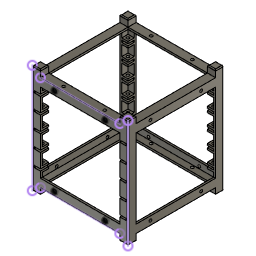
сборка кубсата (Autodesk Fusion 360 archive; units mm, degrees)
design "кубсат 3"
Autodesk Fusion 360 part; units mm, degrees
(part 1 of 2)
sketch "Sketch1" plane through (0, 0, 0) normal (0, 0, 1) x (1, 0, 0)
  line L0 (0, 0) -> (8.5, 0)
  line L1 (8.5, 0) -> (8.5, 8.5)
  line L2 (8.5, 8.5) -> (0, 8.5)
  line L3 (0, 8.5) -> (0, 0)
  line L4 (0, 100) -> (8.5, 100)
  line L5 (8.5, 100) -> (8.5, 91.5)
  line L6 (8.5, 91.5) -> (0, 91.5)
  line L7 (0, 91.5) -> (0, 100)
  line L8 (100, 100) -> (91.5, 100)
  line L9 (91.5, 100) -> (91.5, 91.5)
  line L10 (91.5, 91.5) -> (100, 91.5)
  line L11 (100, 91.5) -> (100, 100)
  line L12 (100, 0) -> (91.5, 0)
  line L13 (91.5, 0) -> (91.5, 8.5)
  line L14 (91.5, 8.5) -> (100, 8.5)
  line L15 (100, 8.5) -> (100, 0)
  dimension "d1" = 100
  dimension "d2" = 100
  dimension "d3" = 8.5
  dimension "d4" = 8.5
  dimension "d5" = 8.5
  dimension "d6" = 8.5
  dimension "d7" = 8.5
  dimension "d8" = 8.5
  dimension "d9" = 83
  dimension "d10" = 83
  dimension "d11" = 8.5
  dimension "d12" = 8.5
  constraint horizontal L0
  constraint vertical L1
  constraint horizontal L2
  constraint vertical L3
  constraint coincident L0.start L3.end
  constraint horizontal L4
  constraint vertical L5
  constraint horizontal L6
  constraint vertical L7
  constraint horizontal L8
  constraint vertical L9
  constraint horizontal L10
  constraint vertical L11
  constraint horizontal L12
  constraint vertical L13
  constraint horizontal L14
  constraint vertical L15
  measures "d1" distance of L0.start L12.start
  measures "d2" distance of L0.start L4.start
  measures "d3" distance of L0.start L0.end
  measures "d4" distance of L0.start L2.end
  measures "d5" distance of L4.start L6.end
  measures "d6" distance of L8.start L8.end
  measures "d7" distance of L12.start L12.end
  measures "d8" distance of L12.start L14.end
  measures "d9" distance of L5 L9
  measures "d10" distance of L10 L14
  measures "d11" distance of L8.start L10.end
  measures "d12" distance of L4.start L4.end
extrude "Extrude1" add sketch "Sketch1" along normal blind 113.5 makes body 1 at (0, 5.6667, 37.8333) makes body 2 at (100, 94.3333, 37.8333) makes body 3 at (2.8333, 100, 37.8333) makes body 4 at (97.1667, 0, 37.8333)
ref_plane "WorkPlane1" through (4.25, 91.5, 56.75) normal (0, -1, 0) x (1, 0, 0)
sketch "Sketch2" plane through (4.25, 91.5, 56.75) normal (0, -1, 0) x (1, 0, 0)
  line L0 (4.25, 47.75) -> (-4.25, 47.75)
  line L1 (-4.25, 47.75) -> (-4.25, 49.75)
  line L2 (-4.25, 49.75) -> (4.25, 49.75)
  line L3 (4.25, 49.75) -> (4.25, 47.75)
  line L4 (-4.25, 56.75) -> (4.25, 56.75)
  line L5 (-4.25, -56.75) -> (-4.25, 56.75)
  line L6 (-4.25, -47.75) -> (4.25, -47.75)
  line L7 (4.25, -47.75) -> (4.25, -49.75)
  line L8 (4.25, -49.75) -> (-4.25, -49.75)
  line L9 (-4.25, -49.75) -> (-4.25, -47.75)
  line L10 (4.25, -56.75) -> (-4.25, -56.75)
  line L11 (4.25, -56.75) -> (4.25, 56.75)
  line L12 (87.25, 49.75) -> (95.75, 49.75)
  line L13 (95.75, 49.75) -> (95.75, 47.75)
  line L14 (95.75, 47.75) -> (87.25, 47.75)
  line L15 (87.25, 47.75) -> (87.25, 49.75)
  line L16 (-4.25, 56.75) -> (4.25, 56.75)
  line L17 (87.25, -56.75) -> (87.25, 56.75)
  line L18 (-4.25, -56.75) -> (4.25, -56.75)
  line L19 (95.75, -56.75) -> (95.75, 56.75)
  line L20 (95.75, -49.75) -> (87.25, -49.75)
  line L21 (87.25, -49.75) -> (87.25, -47.75)
  line L22 (87.25, -47.75) -> (95.75, -47.75)
  line L23 (95.75, -47.75) -> (95.75, -49.75)
  line L24 (95.75, -36.84) -> (87.25, -36.84)
  line L25 (87.25, -36.84) -> (87.25, -34.84)
  line L26 (87.25, -34.84) -> (95.75, -34.84)
  line L27 (95.75, -34.84) -> (95.75, -36.84)
  line L28 (95.75, -32.84) -> (87.25, -32.84)
  line L29 (87.25, -32.84) -> (87.25, -30.84)
  line L30 (87.25, -30.84) -> (95.75, -30.84)
  line L31 (95.75, -30.84) -> (95.75, -32.84)
  line L32 (95.75, -19.93) -> (87.25, -19.93)
  line L33 (87.25, -19.93) -> (87.25, -17.93)
  line L34 (87.25, -17.93) -> (95.75, -17.93)
  line L35 (95.75, -17.93) -> (95.75, -19.93)
  line L36 (95.75, -13.93) -> (87.25, -13.93)
  line L37 (87.25, -13.93) -> (87.25, -15.93)
  line L38 (87.25, -15.93) -> (95.75, -15.93)
  line L39 (95.75, -15.93) -> (95.75, -13.93)
  line L40 (95.75, -3.02) -> (87.25, -3.02)
  line L41 (87.25, -3.02) -> (87.25, -1.02)
  line L42 (87.25, -1.02) -> (95.75, -1.02)
  line L43 (95.75, -1.02) -> (95.75, -3.02)
  line L44 (95.75, 0.98) -> (87.25, 0.98)
  line L45 (87.25, 0.98) -> (87.25, 2.98)
  line L46 (87.25, 2.98) -> (95.75, 2.98)
  line L47 (95.75, 2.98) -> (95.75, 0.98)
  line L48 (95.75, 13.89) -> (87.25, 13.89)
  line L49 (87.25, 13.89) -> (87.25, 15.89)
  line L50 (87.25, 15.89) -> (95.75, 15.89)
  line L51 (95.75, 15.89) -> (95.75, 13.89)
  line L52 (95.75, 17.89) -> (87.25, 17.89)
  line L53 (87.25, 17.89) -> (87.25, 19.89)
  line L54 (87.25, 19.89) -> (95.75, 19.89)
  line L55 (95.75, 19.89) -> (95.75, 17.89)
  line L56 (95.75, 49.75) -> (93.75, 49.75)
  line L57 (93.75, 49.75) -> (93.75, -49.75)
  line L58 (93.75, -49.75) -> (95.75, -49.75)
  line L59 (95.75, -49.75) -> (95.75, 49.75)
  line L60 (95.75, 30.8) -> (87.25, 30.8)
  line L61 (87.25, 30.8) -> (87.25, 32.8)
  line L62 (87.25, 32.8) -> (95.75, 32.8)
  line L63 (95.75, 32.8) -> (95.75, 30.8)
  line L64 (95.75, 34.8) -> (87.25, 34.8)
  line L65 (87.25, 34.8) -> (87.25, 36.8)
  line L66 (87.25, 36.8) -> (95.75, 36.8)
  line L67 (95.75, 36.8) -> (95.75, 34.8)
  line L68 (4.25, -36.84) -> (-4.25, -36.84)
  line L69 (-4.25, -36.84) -> (-4.25, -34.84)
  line L70 (-4.25, -34.84) -> (4.25, -34.84)
  line L71 (4.25, -34.84) -> (4.25, -36.84)
  line L72 (4.25, -32.84) -> (-4.25, -32.84)
  line L73 (-4.25, -32.84) -> (-4.25, -30.84)
  line L74 (-4.25, -30.84) -> (4.25, -30.84)
  line L75 (4.25, -30.84) -> (4.25, -32.84)
  line L76 (4.25, -19.93) -> (-4.25, -19.93)
  line L77 (-4.25, -19.93) -> (-4.25, -17.93)
  line L78 (-4.25, -17.93) -> (4.25, -17.93)
  line L79 (4.25, -17.93) -> (4.25, -19.93)
  line L80 (4.25, -15.93) -> (-4.25, -15.93)
  line L81 (-4.25, -15.93) -> (-4.25, -13.93)
  line L82 (-4.25, -13.93) -> (4.25, -13.93)
  line L83 (4.25, -13.93) -> (4.25, -15.93)
  line L84 (4.25, -3.02) -> (-4.25, -3.02)
  line L85 (-4.25, -3.02) -> (-4.25, -1.02)
  line L86 (-4.25, -1.02) -> (4.25, -1.02)
  line L87 (4.25, -1.02) -> (4.25, -3.02)
  line L88 (4.25, 0.98) -> (-4.25, 0.98)
  line L89 (-4.25, 0.98) -> (-4.25, 2.98)
  line L90 (-4.25, 2.98) -> (4.25, 2.98)
  line L91 (4.25, 2.98) -> (4.25, 0.98)
  line L92 (4.25, 13.89) -> (-4.25, 13.89)
  line L93 (-4.25, 13.89) -> (-4.25, 15.89)
  line L94 (-4.25, 15.89) -> (4.25, 15.89)
  line L95 (4.25, 15.89) -> (4.25, 13.89)
  line L96 (4.25, 17.89) -> (-4.25, 17.89)
  line L97 (-4.25, 17.89) -> (-4.25, 19.89)
  line L98 (-4.25, 19.89) -> (4.25, 19.89)
  line L99 (4.25, 19.89) -> (4.25, 17.89)
  line L100 (4.25, 30.8) -> (-4.25, 30.8)
  line L101 (-4.25, 30.8) -> (-4.25, 32.8)
  line L102 (-4.25, 32.8) -> (4.25, 32.8)
  line L103 (4.25, 32.8) -> (4.25, 30.8)
  line L104 (4.25, 34.8) -> (-4.25, 34.8)
  line L105 (-4.25, 34.8) -> (-4.25, 36.8)
  line L106 (-4.25, 36.8) -> (4.25, 36.8)
  line L107 (4.25, 36.8) -> (4.25, 34.8)
  line L108 (-4.25, 49.75) -> (-2.25, 49.75)
  line L109 (-2.25, 49.75) -> (-2.25, -49.75)
  line L110 (-2.25, -49.75) -> (-4.25, -49.75)
  line L111 (-4.25, -49.75) -> (-4.25, 49.75)
  line L112 (95.75, -56.75) -> (87.25, -56.75)
  line L113 (-2.25, 49.75) -> (-4.25, 49.75)
  line L114 (-4.25, 49.75) -> (-4.25, 41.25)
  line L115 (-4.25, 41.25) -> (-2.25, 41.25)
  line L116 (-2.25, 41.25) -> (-2.25, 49.75)
  line L117 (-4.25, -49.75) -> (-2.25, -49.75)
  line L118 (-2.25, -49.75) -> (-2.25, -41.25)
  line L119 (-2.25, -41.25) -> (-4.25, -41.25)
  line L120 (-4.25, -41.25) -> (-4.25, -49.75)
  line L121 (95.75, -49.75) -> (93.75, -49.75)
  line L122 (93.75, -49.75) -> (93.75, -41.25)
  line L123 (93.75, -41.25) -> (95.75, -41.25)
  line L124 (95.75, -41.25) -> (95.75, -49.75)
  line L125 (95.75, 49.75) -> (93.75, 49.75)
  line L126 (93.75, 49.75) -> (93.75, 41.25)
  line L127 (93.75, 41.25) -> (95.75, 41.25)
  line L128 (95.75, 41.25) -> (95.75, 49.75)
  dimension "d16" = 7
  dimension "d17" = 2
  dimension "d18" = 8.5
  dimension "d19" = 7
  dimension "d20" = 2
  dimension "d21" = 8.5
  dimension "d22" = 7
  dimension "d23" = 2
  dimension "d24" = 8.5
  dimension "d93" = 2
  dimension "d94" = 2
  dimension "d95" = 2
  dimension "d96" = 2
  dimension "d97" = 10.91
  dimension "d98" = 10.91
  dimension "d99" = 2
  dimension "d100" = 2
  dimension "d101" = 2
  dimension "d102" = 10.91
  dimension "d103" = 2
  dimension "d104" = 2
  dimension "d105" = 2
  dimension "d106" = 2
  dimension "d107" = 10.91
  dimension "d108" = 2
  dimension "d109" = 2
  dimension "d111" = 2
  dimension "d112" = 10.91
  dimension "d113" = 2
  dimension "d114" = 2
  dimension "d115" = 2
  dimension "d118" = 10.91
  dimension "d119" = 2
  dimension "d120" = 2
  dimension "d121" = 2
  dimension "d122" = 10.91
  dimension "d123" = 2
  dimension "d124" = 2
  dimension "d125" = 2
  dimension "d126" = 10.91
  dimension "d127" = 2
  dimension "d128" = 2
  dimension "d129" = 2
  dimension "d130" = 10.91
  dimension "d131" = 2
  dimension "d132" = 2
  dimension "d133" = 2
  dimension "d134" = 10.91
  dimension "d135" = 2
  dimension "d136" = 2
  dimension "d137" = 2
  dimension "d139" = 2
  dimension "d151" = 7
  dimension "d152" = 7
  dimension "d153" = 7
  dimension "d187" = 8.5
  dimension "d188" = 8.5
  dimension "d189" = 2
  dimension "d190" = 8.5
  dimension "d192" = 2
  dimension "d193" = 8.5
  constraint horizontal L0
  constraint vertical L1
  constraint horizontal L2
  constraint vertical L3
  constraint collinear L1 L5
  constraint horizontal L6
  constraint vertical L7
  constraint horizontal L8
  constraint vertical L9
  constraint collinear L7 L11
  constraint horizontal L12
  constraint vertical L13
  constraint horizontal L14
  constraint vertical L15
  constraint collinear L15 L17
  constraint horizontal L20
  constraint vertical L21
  constraint horizontal L22
  constraint vertical L23
  constraint coincident L17 L21.end
  constraint horizontal L24
  constraint vertical L25
  constraint horizontal L26
  constraint vertical L27
  constraint coincident L17 L25.end
  constraint coincident L19 L24.start
  constraint horizontal L28
  constraint vertical L29
  constraint horizontal L30
  constraint vertical L31
  constraint coincident L19 L28.start
  constraint horizontal L32
  constraint vertical L33
  constraint horizontal L34
  constraint vertical L35
  constraint coincident L17 L33.end
  constraint coincident L19 L32.start
  constraint horizontal L36
  constraint vertical L37
  constraint horizontal L38
  constraint vertical L39
  constraint coincident L17 L37.end
  constraint collinear L17 L29
  constraint collinear L19 L39
  constraint horizontal L40
  constraint vertical L41
  constraint horizontal L42
  constraint vertical L43
  constraint coincident L19 L40.start
  constraint collinear L17 L41
  constraint horizontal L44
  constraint vertical L45
  constraint horizontal L46
  constraint vertical L47
  constraint coincident L17 L45.end
  constraint coincident L19 L44.start
  constraint horizontal L48
  constraint vertical L49
  constraint horizontal L50
  constraint vertical L51
  constraint coincident L17 L49.end
  constraint coincident L19 L48.start
  constraint horizontal L52
  constraint vertical L53
  constraint horizontal L54
  constraint vertical L55
  constraint coincident L17 L53.end
  constraint coincident L19 L52.start
  constraint horizontal L56
  constraint vertical L57
  constraint horizontal L58
  constraint vertical L59
  constraint horizontal L60
  constraint vertical L61
  constraint horizontal L62
  constraint vertical L63
  constraint coincident L17 L61.end
  constraint coincident L19 L60.start
  constraint horizontal L64
  constraint vertical L65
  constraint horizontal L66
  constraint vertical L67
  constraint coincident L17 L65.end
  constraint coincident L19 L64.start
  constraint horizontal L68
  constraint vertical L69
  constraint horizontal L70
  constraint vertical L71
  constraint coincident L5 L69.end
  constraint coincident L11 L68.start
  constraint horizontal L72
  constraint vertical L73
  constraint horizontal L74
  constraint vertical L75
  constraint coincident L5 L73.end
  constraint coincident L11 L72.start
  constraint horizontal L76
  constraint vertical L77
  constraint horizontal L78
  constraint vertical L79
  constraint coincident L5 L77.end
  constraint coincident L11 L76.start
  constraint horizontal L80
  constraint vertical L81
  constraint horizontal L82
  constraint vertical L83
  constraint coincident L5 L81.end
  constraint coincident L11 L80.start
  constraint horizontal L84
  constraint vertical L85
  constraint horizontal L86
  constraint vertical L87
  constraint coincident L5 L85.end
  constraint coincident L11 L84.start
  constraint horizontal L88
  constraint vertical L89
  constraint horizontal L90
  constraint vertical L91
  constraint coincident L5 L89.end
  constraint coincident L11 L88.start
  constraint horizontal L92
  constraint vertical L93
  constraint horizontal L94
  constraint vertical L95
  constraint coincident L5 L93.end
  constraint coincident L11 L92.start
  constraint horizontal L96
  constraint vertical L97
  constraint horizontal L98
  constraint vertical L99
  constraint coincident L5 L97.end
  constraint coincident L11 L96.start
  constraint horizontal L100
  constraint vertical L101
  constraint horizontal L102
  constraint vertical L103
  constraint coincident L5 L101.end
  constraint coincident L11 L100.start
  constraint horizontal L104
  constraint vertical L105
  constraint horizontal L106
  constraint vertical L107
  constraint coincident L5 L105.end
  constraint coincident L11 L104.start
  constraint horizontal L108
  constraint vertical L109
  constraint horizontal L110
  constraint vertical L111
  constraint collinear L23 L59
  constraint horizontal L113
  constraint vertical L114
  constraint horizontal L115
  constraint vertical L116
  constraint collinear L111 L114
  constraint horizontal L117
  constraint vertical L118
  constraint horizontal L119
  constraint vertical L120
  constraint horizontal L121
  constraint vertical L122
  constraint horizontal L123
  constraint vertical L124
  constraint horizontal L125
  constraint vertical L126
  constraint horizontal L127
  constraint vertical L128
  constraint coincident L57 L126.end
  measures "d16" distance of L2 L4
  measures "d17" distance of L0 L2
  measures "d18" distance of L1 L3
  measures "d19" distance of L8 L10
  measures "d20" distance of L6 L8
  measures "d21" distance of L7 L9
  measures "d22" distance of L12 L16
  measures "d23" distance of L12 L14
  measures "d24" distance of L13 L15
  measures "d93" distance of L20.start L22.end
  measures "d94" distance of L24.start L26.end
  measures "d95" distance of L26 L28
  measures "d96" distance of L28.start L30.end
  measures "d97" distance of L22 L24
  measures "d98" distance of L30 L32
  measures "d99" distance of L32 L34
  measures "d100" distance of L34 L38
  measures "d101" distance of L36 L38
  measures "d102" distance of L36 L40
  measures "d103" distance of L40 L42
  measures "d104" distance of L42 L44
  measures "d105" distance of L44 L46
  measures "d106" distance of L48 L50
  measures "d107" distance of L46 L48
  measures "d108" distance of L50 L52
  measures "d109" distance of L52 L54
  measures "d111" distance of L12.end L56.end
  measures "d112" distance of L54 L60
  measures "d113" distance of L60 L62
  measures "d114" distance of L62 L64
  measures "d115" distance of L64 L66
  measures "d118" distance of L6 L68
  measures "d119" distance of L68.end L69.end
  measures "d120" distance of L70 L72
  measures "d121" distance of L72 L74
  measures "d122" distance of L74 L76
  measures "d123" distance of L76 L78
  measures "d124" distance of L78 L80
  measures "d125" distance of L80 L82
  measures "d126" distance of L82 L84
  measures "d127" distance of L84 L86
  measures "d128" distance of L86 L88
  measures "d129" distance of L88 L90
  measures "d130" distance of L90 L92
  measures "d131" distance of L92 L94
  measures "d132" distance of L94 L96
  measures "d133" distance of L96 L98
  measures "d134" distance of L98 L100
  measures "d135" distance of L100 L102
  measures "d136" distance of L102 L104
  measures "d137" distance of L104 L106
  measures "d139" distance of L1.end L108.end
  measures "d151" distance of L18 L110
  measures "d152" distance of L20 L112
  measures "d153" distance of L58 L112
  measures "d187" distance of L108.end L115.end
  measures "d188" distance of L8.end L119.end
  measures "d189" distance of L118.end L119.end
  measures "d190" distance of L20.start L123.end
  measures "d192" distance of L20.start L57.end
  measures "d193" distance of L12.end L127.end
extrude "Extrude2" add sketch "Sketch2" along normal blind 83 contours L0 L2 L3 L11 L109 L116 | L0 L5 L109 L111 L114 L115 L116 | L0 L1 L2 L5 L108 L109 L111 L113 L114 L116 | L6 L7 L8 L11 L109 L118 | L5 L6 L8 L9 L109 L110 L111 L117 L118 L120 | L5 L6 L109 L111 L118 L119 L120 | L12 L14 L15 L17 L57 L126 | L12 L13 L14 L19 L56 L57 L59 L125 L126 L128 | L14 L19 L57 L59 L126 L127 L128 | L17 L20 L21 L22 L57 L122 | L19 L22 L57 L59 L122 L123 L124 | L19 L20 L22 L23 L57 L58 L59 L121 L122 L124 bodies 1 2 3 4
ref_plane "WorkPlane2" through (91.5, 50, 56.75) normal (-1, 0, 0) x (0, -1, 0)
sketch "Sketch3" plane through (91.5, 50, 56.75) normal (-1, 0, 0) x (0, 1, 0)
  line L0 (50, -49.75) -> (48, -49.75)
  line L1 (48, -49.75) -> (48, 49.75)
  line L2 (48, 49.75) -> (50, 49.75)
  line L3 (50, 49.75) -> (50, -49.75)
  line L4 (50, -56.75) -> (41.5, -56.75)
  line L5 (50, 56.75) -> (50, -56.75)
  line L6 (41.5, 56.75) -> (50, 56.75)
  line L7 (-41.5, 47.75) -> (-50, 47.75)
  line L8 (-50, 47.75) -> (-50, 49.75)
  line L9 (-50, 49.75) -> (-41.5, 49.75)
  line L10 (-41.5, 49.75) -> (-41.5, 47.75)
  line L11 (-41.5, 56.75) -> (-50, 56.75)
  line L12 (-41.5, 56.75) -> (-41.5, 49.75)
  line L13 (-41.5, -56.75) -> (-50, -56.75)
  line L14 (50, -49.75) -> (41.5, -49.75)
  line L15 (41.5, -49.75) -> (41.5, -47.75)
  line L16 (41.5, -47.75) -> (50, -47.75)
  line L17 (50, -47.75) -> (50, -49.75)
  line L18 (50, -36.84) -> (41.5, -36.84)
  line L19 (41.5, -36.84) -> (41.5, -34.84)
  line L20 (41.5, -34.84) -> (50, -34.84)
  line L21 (50, -34.84) -> (50, -36.84)
  line L22 (50, -32.84) -> (41.5, -32.84)
  line L23 (41.5, -32.84) -> (41.5, -30.84)
  line L24 (41.5, -30.84) -> (50, -30.84)
  line L25 (50, -30.84) -> (50, -32.84)
  line L26 (41.5, 41.25) -> (41.5, -41.25)
  line L27 (50, -19.93) -> (41.5, -19.93)
  line L28 (41.5, -19.93) -> (41.5, -17.93)
  line L29 (41.5, -17.93) -> (50, -17.93)
  line L30 (50, -17.93) -> (50, -19.93)
  line L31 (50, -15.93) -> (41.5, -15.93)
  line L32 (41.5, -15.93) -> (41.5, -13.93)
  line L33 (41.5, -13.93) -> (50, -13.93)
  line L34 (50, -13.93) -> (50, -15.93)
  line L35 (50, -3.02) -> (41.5, -3.02)
  line L36 (41.5, -3.02) -> (41.5, -1.02)
  line L37 (41.5, -1.02) -> (50, -1.02)
  line L38 (50, -1.02) -> (50, -3.02)
  line L39 (50, 0.98) -> (41.5, 0.98)
  line L40 (41.5, 0.98) -> (41.5, 2.98)
  line L41 (41.5, 2.98) -> (50, 2.98)
  line L42 (50, 2.98) -> (50, 0.98)
  line L43 (50, 13.89) -> (41.5, 13.89)
  line L44 (41.5, 13.89) -> (41.5, 15.89)
  line L45 (41.5, 15.89) -> (50, 15.89)
  line L46 (50, 15.89) -> (50, 13.89)
  line L47 (50, 17.89) -> (41.5, 17.89)
  line L48 (41.5, 17.89) -> (41.5, 19.89)
  line L49 (41.5, 19.89) -> (50, 19.89)
  line L50 (50, 19.89) -> (50, 17.89)
  line L51 (50, 30.8) -> (41.5, 30.8)
  line L52 (41.5, 30.8) -> (41.5, 32.8)
  line L53 (41.5, 32.8) -> (50, 32.8)
  line L54 (50, 32.8) -> (50, 30.8)
  line L55 (50, 34.8) -> (41.5, 34.8)
  line L56 (41.5, 34.8) -> (41.5, 36.8)
  line L57 (41.5, 36.8) -> (50, 36.8)
  line L58 (50, 36.8) -> (50, 34.8)
  line L59 (50, 49.75) -> (41.5, 49.75)
  line L60 (41.5, 49.75) -> (41.5, 47.75)
  line L61 (41.5, 47.75) -> (50, 47.75)
  line L62 (50, 47.75) -> (50, 49.75)
  line L63 (41.5, 56.75) -> (41.5, 49.75)
  line L64 (-41.5, -36.84) -> (-50, -36.84)
  line L65 (-50, -36.84) -> (-50, -34.84)
  line L66 (-50, -34.84) -> (-41.5, -34.84)
  line L67 (-41.5, -34.84) -> (-41.5, -36.84)
  line L68 (-50, 56.75) -> (-50, -56.75)
  line L69 (-41.5, -32.84) -> (-50, -32.84)
  line L70 (-50, -32.84) -> (-50, -30.84)
  line L71 (-50, -30.84) -> (-41.5, -30.84)
  line L72 (-41.5, -30.84) -> (-41.5, -32.84)
  line L73 (-41.5, -19.93) -> (-50, -19.93)
  line L74 (-50, -19.93) -> (-50, -17.93)
  line L75 (-50, -17.93) -> (-41.5, -17.93)
  line L76 (-41.5, -17.93) -> (-41.5, -19.93)
  line L77 (-41.5, -15.93) -> (-50, -15.93)
  line L78 (-50, -15.93) -> (-50, -13.93)
  line L79 (-50, -13.93) -> (-41.5, -13.93)
  line L80 (-41.5, -13.93) -> (-41.5, -15.93)
  line L81 (-41.5, -3.02) -> (-50, -3.02)
  line L82 (-50, -3.02) -> (-50, -1.02)
  line L83 (-50, -1.02) -> (-41.5, -1.02)
  line L84 (-41.5, -1.02) -> (-41.5, -3.02)
  line L85 (-41.5, 0.98) -> (-50, 0.98)
  line L86 (-50, 0.98) -> (-50, 2.98)
  line L87 (-50, 2.98) -> (-41.5, 2.98)
  line L88 (-41.5, 2.98) -> (-41.5, 0.98)
  line L89 (-41.5, 13.89) -> (-50, 13.89)
  line L90 (-50, 13.89) -> (-50, 15.89)
  line L91 (-50, 15.89) -> (-41.5, 15.89)
  line L92 (-41.5, 15.89) -> (-41.5, 13.89)
  line L93 (-41.5, 17.89) -> (-50, 17.89)
  line L94 (-50, 17.89) -> (-50, 19.89)
  line L95 (-50, 19.89) -> (-41.5, 19.89)
  line L96 (-41.5, 19.89) -> (-41.5, 17.89)
  line L97 (-41.5, 30.8) -> (-50, 30.8)
  line L98 (-50, 30.8) -> (-50, 32.8)
  line L99 (-50, 32.8) -> (-41.5, 32.8)
  line L100 (-41.5, 32.8) -> (-41.5, 30.8)
  line L101 (-41.5, 34.8) -> (-50, 34.8)
  line L102 (-50, 34.8) -> (-50, 36.8)
  line L103 (-50, 36.8) -> (-41.5, 36.8)
  line L104 (-41.5, 36.8) -> (-41.5, 34.8)
  line L105 (-41.5, -49.75) -> (-50, -49.75)
  line L106 (-50, -49.75) -> (-50, -47.75)
  line L107 (-50, -47.75) -> (-41.5, -47.75)
  line L108 (-41.5, -47.75) -> (-41.5, -49.75)
  line L109 (-50, -49.75) -> (-48, -49.75)
  line L110 (-48, -49.75) -> (-48, 49.75)
  line L111 (-48, 49.75) -> (-50, 49.75)
  line L112 (-50, 49.75) -> (-50, -49.75)
  line L113 (-41.5, 41.25) -> (-41.5, -41.25)
  line L114 (-41.5, -49.75) -> (-41.5, -56.75)
  line L115 (41.5, -49.75) -> (41.5, -56.75)
  line L116 (41.5, 56.75) -> (41.5, 49.75)
  line L117 (50, -49.75) -> (48, -49.75)
  line L118 (48, -49.75) -> (48, -41.25)
  line L119 (48, -41.25) -> (50, -41.25)
  line L120 (50, -41.25) -> (50, -49.75)
  line L121 (50, 49.75) -> (48, 49.75)
  line L122 (48, 49.75) -> (48, 41.25)
  line L123 (48, 41.25) -> (50, 41.25)
  line L124 (50, 41.25) -> (50, 49.75)
  line L125 (-50, 49.75) -> (-48, 49.75)
  line L126 (-48, 49.75) -> (-48, 41.25)
  line L127 (-48, 41.25) -> (-50, 41.25)
  line L128 (-50, 41.25) -> (-50, 49.75)
  line L129 (-50, -49.75) -> (-48, -49.75)
  line L130 (-48, -49.75) -> (-48, -41.25)
  line L131 (-48, -41.25) -> (-50, -41.25)
  line L132 (-50, -41.25) -> (-50, -49.75)
  line L133 (-48, 47.75) -> (-41.5, 47.75)
  line L134 (-41.5, 47.75) -> (-41.5, 36.8)
  line L135 (-41.5, 36.8) -> (-48, 36.8)
  line L136 (-48, 36.8) -> (-48, 47.75)
  dimension "d31" = 7
  dimension "d33" = 2
  dimension "d37" = 7
  dimension "d38" = 2
  dimension "d39" = 8.5
  dimension "d45" = 2
  dimension "d46" = 8.5
  dimension "d47" = 10.91
  dimension "d48" = 2
  dimension "d49" = 2
  dimension "d50" = 2
  dimension "d51" = 10.91
  dimension "d52" = 2
  dimension "d53" = 113.5
  dimension "d54" = 2
  dimension "d55" = 2
  dimension "d56" = 2
  dimension "d57" = 10.91
  dimension "d58" = 2
  dimension "d59" = 2
  dimension "d60" = 10.91
  dimension "d61" = 2
  dimension "d62" = 2
  dimension "d63" = 2
  dimension "d64" = 10.91
  dimension "d65" = 2
  dimension "d66" = 2
  dimension "d67" = 2
  dimension "d68" = 2
  dimension "d71" = 2
  dimension "d73" = 2
  dimension "d74" = 2
  dimension "d75" = 2
  dimension "d76" = 10.91
  dimension "d77" = 2
  dimension "d78" = 2
  dimension "d79" = 10.91
  dimension "d80" = 2
  dimension "d81" = 2
  dimension "d82" = 2
  dimension "d83" = 10.91
  dimension "d84" = 2
  dimension "d85" = 2
  dimension "d86" = 2
  dimension "d87" = 10.91
  dimension "d88" = 2
  dimension "d89" = 2
  dimension "d90" = 2
  dimension "d141" = 2
  dimension "d142" = 8.5
  dimension "d143" = 7
  dimension "d144" = 10.91
  dimension "d146" = 2
  dimension "d147" = 7
  dimension "d148" = 7
  dimension "d149" = 8.5
  dimension "d150" = 7
  dimension "d194" = 8.5
  dimension "d195" = 8.5
  dimension "d196" = 2
  dimension "d197" = 8.5
  dimension "d198" = 2
  dimension "d199" = 8.5
  dimension "d200" = 2
  constraint horizontal L0
  constraint vertical L1
  constraint horizontal L2
  constraint vertical L3
  constraint collinear L3 L5
  constraint horizontal L7
  constraint vertical L8
  constraint horizontal L9
  constraint vertical L10
  constraint collinear L10 L12
  constraint horizontal L14
  constraint vertical L15
  constraint horizontal L16
  constraint vertical L17
  constraint horizontal L18
  constraint vertical L19
  constraint horizontal L20
  constraint vertical L21
  constraint coincident L5 L18.start
  constraint horizontal L22
  constraint vertical L23
  constraint horizontal L24
  constraint vertical L25
  constraint coincident L5 L22.start
  constraint collinear L19 L26
  constraint collinear L23 L26
  constraint horizontal L27
  constraint vertical L28
  constraint horizontal L29
  constraint vertical L30
  constraint horizontal L31
  constraint vertical L32
  constraint horizontal L33
  constraint vertical L34
  constraint coincident L5 L31.start
  constraint collinear L26 L28
  constraint collinear L5 L30
  constraint collinear L26 L32
  constraint horizontal L35
  constraint vertical L36
  constraint horizontal L37
  constraint vertical L38
  constraint coincident L26 L36.end
  constraint coincident L5 L35.start
  constraint horizontal L39
  constraint vertical L40
  constraint horizontal L41
  constraint vertical L42
  constraint coincident L5 L39.start
  constraint horizontal L43
  constraint vertical L44
  constraint horizontal L45
  constraint vertical L46
  constraint collinear L26 L40
  constraint horizontal L47
  constraint vertical L48
  constraint horizontal L49
  constraint vertical L50
  constraint collinear L5 L46
  constraint collinear L26 L44
  constraint collinear L26 L48
  constraint collinear L5 L50
  constraint horizontal L51
  constraint vertical L52
  constraint horizontal L53
  constraint vertical L54
  constraint coincident L26 L52.end
  constraint coincident L5 L51.start
  constraint horizontal L55
  constraint vertical L56
  constraint horizontal L57
  constraint vertical L58
  constraint coincident L26 L56.end
  constraint coincident L5 L55.start
  constraint horizontal L59
  constraint vertical L60
  constraint horizontal L61
  constraint vertical L62
  constraint collinear L60 L63
  constraint horizontal L64
  constraint vertical L65
  constraint horizontal L66
  constraint vertical L67
  constraint coincident L12 L64.start
  constraint collinear L65 L68
  constraint horizontal L69
  constraint vertical L70
  constraint horizontal L71
  constraint vertical L72
  constraint coincident L12 L69.start
  constraint collinear L68 L70
  constraint horizontal L73
  constraint vertical L74
  constraint horizontal L75
  constraint vertical L76
  constraint coincident L12 L73.start
  constraint horizontal L77
  constraint vertical L78
  constraint horizontal L79
  constraint vertical L80
  constraint coincident L68 L78.end
  constraint coincident L12 L77.start
  constraint collinear L68 L74
  constraint horizontal L81
  constraint vertical L82
  constraint horizontal L83
  constraint vertical L84
  constraint coincident L68 L82.end
  constraint coincident L12 L81.start
  constraint horizontal L85
  constraint vertical L86
  constraint horizontal L87
  constraint vertical L88
  constraint coincident L68 L86.end
  constraint coincident L12 L85.start
  constraint horizontal L89
  constraint vertical L90
  constraint horizontal L91
  constraint vertical L92
  constraint coincident L12 L89.start
  constraint horizontal L93
  constraint vertical L94
  constraint horizontal L95
  constraint vertical L96
  constraint coincident L68 L94.end
  constraint coincident L12 L93.start
  constraint collinear L68 L90
  constraint horizontal L97
  constraint vertical L98
  constraint horizontal L99
  constraint vertical L100
  constraint coincident L12 L97.start
  constraint horizontal L101
  constraint vertical L102
  constraint horizontal L103
  constraint vertical L104
  constraint coincident L68 L102.end
  constraint coincident L12 L101.start
  constraint collinear L68 L98
  constraint horizontal L105
  constraint vertical L106
  constraint horizontal L107
  constraint vertical L108
  constraint coincident L68 L106.end
  constraint horizontal L109
  constraint vertical L110
  constraint horizontal L111
  constraint vertical L112
  constraint horizontal L117
  constraint vertical L118
  constraint horizontal L119
  constraint vertical L120
  constraint coincident L1 L118.end
  constraint horizontal L121
  constraint vertical L122
  constraint horizontal L123
  constraint vertical L124
  constraint horizontal L125
  constraint vertical L126
  constraint horizontal L127
  constraint vertical L128
  constraint horizontal L129
  constraint vertical L130
  constraint horizontal L131
  constraint vertical L132
  constraint horizontal L133
  constraint vertical L134
  constraint horizontal L135
  constraint vertical L136
  constraint coincident L126 L133.start
  constraint coincident L7 L133.start
  measures "d31" distance of L0 L4
  measures "d33" distance of L1 L3
  measures "d37" distance of L9 L11
  measures "d38" distance of L7 L9
  measures "d39" distance of L8 L10
  measures "d45" distance of L14.end L15.end
  measures "d46" distance of L0.start L14.end
  measures "d47" distance of L16 L18
  measures "d48" distance of L18.start L20.end
  measures "d49" distance of L20 L22
  measures "d50" distance of L22 L24
  measures "d51" distance of L24 L27
  measures "d52" distance of L27 L29
  measures "d53" distance of L4.start L5.start
  measures "d54" distance of L31.start L33.end
  measures "d55" distance of L29 L31
  measures "d56" distance of L35.start L37.end
  measures "d57" distance of L33 L35
  measures "d58" distance of L37 L39
  measures "d59" distance of L39 L41
  measures "d60" distance of L41 L43
  measures "d61" distance of L43 L45
  measures "d62" distance of L45 L47
  measures "d63" distance of L47 L49
  measures "d64" distance of L49 L51
  measures "d65" distance of L51.start L53.end
  measures "d66" distance of L55 L57
  measures "d67" distance of L53 L55
  measures "d68" distance of L2.end L61.end
  measures "d71" distance of L64.end L65.end
  measures "d73" distance of L66 L69
  measures "d74" distance of L69 L71
  measures "d75" distance of L73 L75
  measures "d76" distance of L71 L73
  measures "d77" distance of L77.end L78.end
  measures "d78" distance of L75 L77
  measures "d79" distance of L79 L81
  measures "d80" distance of L81.end L82.end
  measures "d81" distance of L83 L85
  measures "d82" distance of L85 L87
  measures "d83" distance of L87 L89
  measures "d84" distance of L89.end L90.end
  measures "d85" distance of L91 L93
  measures "d86" distance of L93 L95
  measures "d87" distance of L95 L97
  measures "d88" distance of L97 L99
  measures "d89" distance of L99 L101
  measures "d90" distance of L101 L103
  measures "d141" distance of L105.end L106.end
  measures "d142" distance of L105.start L105.end
  measures "d143" distance of L13 L105
  measures "d144" distance of L64 L107
  measures "d146" distance of L105.end L109.end
  measures "d147" distance of L11 L111
  measures "d148" distance of L2 L6
  measures "d149" distance of L2.end L59.end
  measures "d150" distance of L6 L59
  measures "d194" distance of L0.start L119.end
  measures "d195" distance of L2.end L123.end
  measures "d196" distance of L2.end L1.end
  measures "d197" distance of L8.end L127.end
  measures "d198" distance of L126.end L127.end
  measures "d199" distance of L105.end L131.end
  measures "d200" distance of L105.end L109.end
extrude "Extrude3" add sketch "Sketch3" along normal blind 83 contours L0 L1 L3 L5 L14 L16 L17 L117 L118 L120 | L1 L14 L15 L16 L118 | L1 L3 L5 L16 L118 L119 L120 | L1 L3 L5 L61 L122 L123 L124 | L1 L2 L3 L5 L59 L61 L62 L121 L122 L124 | L1 L59 L60 L61 L122 | L7 L9 L10 L110 L126 L133 | L7 L68 L110 L112 L126 L127 L128 L136 | L7 L8 L9 L68 L110 L111 L112 L125 L126 L128 | L68 L107 L110 L112 L130 L131 L132 | L68 L105 L106 L107 L109 L110 L112 L129 L130 L132 | L105 L107 L108 L110 L130 bodies 1 2
extrude "Extrude4" cut sketch "Sketch2" against normal blind 6.5 contours L0 L11 L106 L109 L116 | L11 L102 L104 L109 | L11 L98 L100 L109 | L11 L94 L96 L109 | L11 L90 L92 L109 | L11 L86 L88 L109 | L11 L82 L84 L109 | L11 L78 L80 L109 | L11 L74 L76 L109 | L11 L70 L72 L109 | L6 L11 L68 L109 L118 | L14 L17 L57 L66 L126 | L17 L57 L62 L64 | L17 L54 L57 L60 | L17 L50 L52 L57 | L17 L46 L48 L57 | L17 L42 L44 L57 | L17 L36 L40 L57 | L17 L34 L38 L57 | L17 L30 L32 L57 | L17 L26 L28 L57 | L17 L22 L24 L57 L122 bodies 1
extrude "Extrude5" cut sketch "Sketch3" against normal blind 6.5 contours L7 L103 L110 L113 L126 L133 L134 L135 L136 | L99 L101 L110 L113 | L68 L99 L101 L110 L112 | L95 L97 L110 L113 | L91 L93 L110 L113 | L68 L91 L93 L110 L112 | L87 L89 L110 L113 | L83 L85 L110 L113 | L68 L83 L85 L110 L112 | L79 L81 L110 L113 | L75 L77 L110 L113 | L68 L75 L77 L110 L112 | L71 L73 L110 L113 | L66 L69 L110 L113 | L66 L68 L69 L110 L112 bodies 1
ref_plane "WorkPlane3" through (8.5, 50, 56.75) normal (1, 0, 0) x (0, 1, 0)
sketch "Sketch4" plane through (8.5, 4.25, 56.75) normal (1, 0, 0) x (0, 1, 0)
  line L0 (-4.25, 49.75) -> (-2.25, 49.75)
  line L1 (-2.25, 49.75) -> (-2.25, -49.75)
  line L2 (-2.25, -49.75) -> (-4.25, -49.75)
  line L3 (-4.25, -49.75) -> (-4.25, 49.75)
  line L4 (-4.25, 56.75) -> (4.25, 56.75)
  line L5 (4.25, -56.75) -> (-4.25, -56.75)
  line L6 (-4.25, -56.75) -> (-4.25, 56.75)
  line L7 (-4.25, 36.84) -> (4.25, 36.84)
  line L8 (4.25, 36.84) -> (4.25, 34.84)
  line L9 (4.25, 34.84) -> (-4.25, 34.84)
  line L10 (-4.25, 34.84) -> (-4.25, 36.84)
  line L11 (4.25, 49.75) -> (4.25, 47.75)
  line L12 (4.25, 47.75) -> (-4.25, 47.75)
  line L13 (-4.25, 47.75) -> (-4.25, 49.75)
  line L14 (4.25, 49.75) -> (4.25, 56.75)
  line L15 (-4.25, 32.84) -> (4.25, 32.84)
  line L16 (4.25, 32.84) -> (4.25, 30.84)
  line L17 (4.25, 30.84) -> (-4.25, 30.84)
  line L18 (-4.25, 30.84) -> (-4.25, 32.84)
  line L19 (-4.25, 19.93) -> (4.25, 19.93)
  line L20 (4.25, 19.93) -> (4.25, 17.93)
  line L21 (4.25, 17.93) -> (-4.25, 17.93)
  line L22 (-4.25, 17.93) -> (-4.25, 19.93)
  line L23 (-4.25, 15.93) -> (4.25, 15.93)
  line L24 (4.25, 15.93) -> (4.25, 13.93)
  line L25 (4.25, 13.93) -> (-4.25, 13.93)
  line L26 (-4.25, 13.93) -> (-4.25, 15.93)
  line L27 (-4.25, 3.02) -> (4.25, 3.02)
  line L28 (4.25, 3.02) -> (4.25, 1.02)
  line L29 (4.25, 1.02) -> (-4.25, 1.02)
  line L30 (-4.25, 1.02) -> (-4.25, 3.02)
  line L31 (-4.25, -0.98) -> (4.25, -0.98)
  line L32 (4.25, -0.98) -> (4.25, -2.98)
  line L33 (4.25, -2.98) -> (-4.25, -2.98)
  line L34 (-4.25, -2.98) -> (-4.25, -0.98)
  line L35 (-4.25, -13.89) -> (4.25, -13.89)
  line L36 (4.25, -13.89) -> (4.25, -15.89)
  line L37 (4.25, -15.89) -> (-4.25, -15.89)
  line L38 (-4.25, -15.89) -> (-4.25, -13.89)
  line L39 (-4.25, -17.89) -> (4.25, -17.89)
  line L40 (4.25, -17.89) -> (4.25, -19.89)
  line L41 (4.25, -19.89) -> (-4.25, -19.89)
  line L42 (-4.25, -19.89) -> (-4.25, -17.89)
  line L43 (-4.25, -30.8) -> (4.25, -30.8)
  line L44 (4.25, -30.8) -> (4.25, -32.8)
  line L45 (4.25, -32.8) -> (-4.25, -32.8)
  line L46 (-4.25, -32.8) -> (-4.25, -30.8)
  line L47 (-4.25, -34.8) -> (4.25, -34.8)
  line L48 (4.25, -34.8) -> (4.25, -36.8)
  line L49 (4.25, -36.8) -> (-4.25, -36.8)
  line L50 (-4.25, -36.8) -> (-4.25, -34.8)
  line L51 (-4.25, -49.75) -> (4.25, -49.75)
  line L52 (4.25, -49.75) -> (4.25, 49.75)
  line L53 (4.25, 49.75) -> (-4.25, 49.75)
  line L54 (-4.25, 49.75) -> (-4.25, -49.75)
  line L55 (4.25, -41.25) -> (4.25, 41.25)
  line L56 (4.25, -56.75) -> (4.25, -49.75)
  line L57 (4.25, 49.75) -> (4.25, 56.75)
  dimension "d159" = 7
  dimension "d160" = 2
  dimension "d161" = 7
  dimension "d164" = 10.91
  dimension "d165" = 2
  dimension "d166" = 2
  dimension "d167" = 2
  dimension "d168" = 10.91
  dimension "d169" = 2
  dimension "d170" = 2
  dimension "d171" = 2
  dimension "d172" = 10.91
  dimension "d173" = 2
  dimension "d174" = 2
  dimension "d175" = 2
  dimension "d176" = 10.91
  dimension "d177" = 2
  dimension "d178" = 2
  dimension "d179" = 2
  dimension "d180" = 10.91
  dimension "d181" = 2
  dimension "d182" = 2
  dimension "d183" = 2
  dimension "d262" = 2
  dimension "d263" = 8.5
  dimension "d264" = 7
  constraint horizontal L0
  constraint vertical L1
  constraint horizontal L2
  constraint vertical L3
  constraint collinear L3 L6
  constraint horizontal L7
  constraint vertical L8
  constraint horizontal L9
  constraint vertical L10
  constraint coincident L6 L7.start
  constraint coincident L3 L7.start
  constraint vertical L11
  constraint horizontal L12
  constraint vertical L13
  constraint collinear L11 L14
  constraint horizontal L15
  constraint vertical L16
  constraint horizontal L17
  constraint vertical L18
  constraint coincident L3 L15.start
  constraint horizontal L19
  constraint vertical L20
  constraint horizontal L21
  constraint vertical L22
  constraint coincident L6 L19.start
  constraint horizontal L23
  constraint vertical L24
  constraint horizontal L25
  constraint vertical L26
  constraint coincident L3 L23.start
  constraint horizontal L27
  constraint vertical L28
  constraint horizontal L29
  constraint vertical L30
  constraint coincident L3 L27.start
  constraint horizontal L31
  constraint vertical L32
  constraint horizontal L33
  constraint vertical L34
  constraint coincident L6 L31.start
  constraint horizontal L35
  constraint vertical L36
  constraint horizontal L37
  constraint vertical L38
  constraint coincident L3 L35.start
  constraint horizontal L39
  constraint vertical L40
  constraint horizontal L41
  constraint vertical L42
  constraint coincident L6 L39.start
  constraint horizontal L43
  constraint vertical L44
  constraint horizontal L45
  constraint vertical L46
  constraint coincident L6 L43.start
  constraint horizontal L47
  constraint vertical L48
  constraint horizontal L49
  constraint vertical L50
  constraint coincident L6 L47.start
  constraint horizontal L51
  constraint vertical L52
  constraint horizontal L53
  constraint vertical L54
  constraint collinear L52 L56
  constraint collinear L8 L52
  constraint collinear L16 L52
  constraint collinear L36 L52
  constraint collinear L40 L52
  constraint collinear L44 L52
  constraint collinear L48 L52
  constraint collinear L24 L52
  constraint collinear L20 L52
  constraint collinear L28 L52
  constraint collinear L32 L52
  measures "d159" distance of L0 L4
  measures "d160" distance of L0.start L0.end
  measures "d161" distance of L2 L5
  measures "d164" distance of L7 L12
  measures "d165" distance of L7 L9
  measures "d166" distance of L9 L15
  measures "d167" distance of L15 L17
  measures "d168" distance of L17 L19
  measures "d169" distance of L19 L21
  measures "d170" distance of L21 L23
  measures "d171" distance of L23 L25
  measures "d172" distance of L25 L27
  measures "d173" distance of L27 L29
  measures "d174" distance of L29 L31
  measures "d175" distance of L31 L33
  measures "d176" distance of L33 L35
  measures "d177" distance of L35 L37
  measures "d178" distance of L37 L39
  measures "d179" distance of L39 L41
  measures "d180" distance of L41 L43
  measures "d181" distance of L43 L45
  measures "d182" distance of L45 L47
  measures "d183" distance of L47 L49
  measures "d262" distance of L12 L53
  measures "d263" distance of L11.start L0.start
  measures "d264" distance of L4 L53
extrude "Extrude6" cut sketch "Sketch4" against normal blind 6.5 contours L1 L7 L12 L52 L55 | L1 L3 L6 L9 L15 L54 | L1 L9 L15 L52 L55 | L1 L17 L19 L52 L55 | L1 L3 L6 L21 L23 L54 | L1 L21 L23 L52 L55 | L1 L25 L27 L52 L55 | L1 L3 L6 L29 L31 L54 | L1 L29 L31 L52 L55 | L1 L33 L35 L52 L55 | L1 L3 L6 L37 L39 L54 | L1 L37 L39 L52 L55 | L1 L41 L43 L52 L55 | L1 L3 L6 L45 L47 L54 | L1 L45 L47 L52 L55 | L1 L49 L51 L52 L55 bodies 1
ref_plane "WorkPlane4" through (5.25, 5.25, 93.59) normal (0, 0, 1) x (0, 1, 0)
sketch "Sketch5" plane through (5.25, 5.25, 93.59) normal (0, 0, 1) x (1, 0, 0)
  line L0 (3.25, 3.25) -> (-3.25, 3.25)
  line L1 (-3.25, 3.25) -> (-3.25, -3.25)
  line L2 (-3.25, -3.25) -> (3.25, -3.25)
  line L3 (3.25, -3.25) -> (3.25, 3.25)
  line L4 (3.25, -5.25) -> (3.25, 3.25)
  line L5 (3.25, 3.25) -> (-5.25, 3.25)
  circle A0 centre (0, 0) radius 1.465
  line L6 (3.25, 86.25) -> (-3.25, 86.25)
  line L7 (-3.25, 86.25) -> (-3.25, 92.75)
  line L8 (-3.25, 92.75) -> (3.25, 92.75)
  line L9 (3.25, 92.75) -> (3.25, 86.25)
  line L10 (-5.25, 86.25) -> (3.25, 86.25)
  line L11 (3.25, 86.25) -> (3.25, 94.75)
  circle A1 centre (0, 89.5) radius 1.465
  line L12 (86.25, 86.25) -> (92.75, 86.25)
  line L13 (92.75, 86.25) -> (92.75, 92.75)
  line L14 (92.75, 92.75) -> (86.25, 92.75)
  line L15 (86.25, 92.75) -> (86.25, 86.25)
  line L16 (86.25, 94.75) -> (86.25, 86.25)
  line L17 (86.25, 86.25) -> (94.75, 86.25)
  circle A2 centre (89.5, 89.5) radius 1.465
  line L18 (92.75, -3.25) -> (86.25, -3.25)
  line L19 (86.25, -3.25) -> (86.25, 3.25)
  line L20 (86.25, 3.25) -> (92.75, 3.25)
  line L21 (92.75, 3.25) -> (92.75, -3.25)
  line L22 (94.75, 3.25) -> (86.25, 3.25)
  line L23 (86.25, 3.25) -> (86.25, -5.25)
  circle A3 centre (89.5, 0) radius 1.465
  dimension "d201" = 6.5
  dimension "d202" = 6.5
  dimension "d203" = 2.93
  dimension "d204" = 6.5
  dimension "d205" = 6.5
  dimension "d206" = 2.93
  dimension "d207" = 3.25
  dimension "d208" = 3.25
  dimension "d209" = 6.5
  dimension "d210" = 6.5
  dimension "d211" = 2.93
  dimension "d212" = 3.25
  dimension "d213" = 3.25
  dimension "d214" = 6.5
  dimension "d215" = 6.5
  dimension "d216" = 2.93
  dimension "d217" = 3.25
  dimension "d218" = 3.25
  constraint horizontal L0
  constraint vertical L1
  constraint horizontal L2
  constraint vertical L3
  constraint collinear L3 L4
  constraint collinear L0 L5
  constraint coincident A0.centre origin
  constraint horizontal L6
  constraint vertical L7
  constraint horizontal L8
  constraint vertical L9
  constraint collinear L6 L10
  constraint collinear L9 L11
  constraint horizontal L12
  constraint vertical L13
  constraint horizontal L14
  constraint vertical L15
  constraint collinear L15 L16
  constraint collinear L12 L17
  constraint horizontal L18
  constraint vertical L19
  constraint horizontal L20
  constraint vertical L21
  constraint collinear L20 L22
  constraint collinear L19 L23
  measures "d201" distance of L0.start L0.end
  measures "d202" distance of L0.start L2.end
  measures "d203" diameter of A0
  measures "d204" distance of L6.start L6.end
  measures "d205" distance of L6.start L8.end
  measures "d206" diameter of A1
  measures "d207" distance of L9 A1.centre
  measures "d208" distance of L6 A1.centre
  measures "d209" distance of L12.start L12.end
  measures "d210" distance of L12.start L14.end
  measures "d211" diameter of A2
  measures "d212" distance of L15 A2.centre
  measures "d213" distance of L12 A2.centre
  measures "d214" distance of L18.start L18.end
  measures "d215" distance of L18.start L20.end
  measures "d216" diameter of A3
  measures "d217" distance of L20 A3.centre
  measures "d218" distance of L19 A3.centre
extrude "Extrude7" cut sketch "Sketch5" against normal blind 74 contours A0 | A1 | A2 | A3 bodies 1
ref_plane "WorkPlane5" through (50, 4.25, 106.5) normal (0, 0, 1) x (0, 1, 0)
sketch "Sketch6" plane through (50, 4.25, 106.5) normal (0, 0, 1) x (1, 0, 0)
  circle A0 centre (-21.5, 0) radius 1.465
  circle A1 centre (21.5, 0) radius 1.465
  line L0 (41.5, 4.25) -> (-41.5, 4.25)
  line L1 (-41.5, -4.25) -> (-41.5, 4.25)
  line L2 (41.5, 4.25) -> (41.5, -4.25)
  line L3 (41.5, 87.25) -> (41.5, 4.25)
  line L4 (50, 4.25) -> (41.5, 4.25)
  line L5 (41.5, 87.25) -> (50, 87.25)
  circle A2 centre (21.5, 91.5) radius 1.465
  line L6 (41.5, 87.25) -> (-41.5, 87.25)
  line L7 (41.5, 95.75) -> (41.5, 87.25)
  circle A3 centre (-21.5, 91.5) radius 1.465
  line L8 (41.5, 95.75) -> (-41.5, 95.75)
  line L9 (-41.5, 87.25) -> (-41.5, 95.75)
  line L10 (-41.5, 87.25) -> (-41.5, 4.25)
  line L11 (-50, 87.25) -> (-41.5, 87.25)
  line L12 (-41.5, 4.25) -> (-50, 4.25)
  dimension "d222" = 2.93
  dimension "d223" = 2.93
  dimension "d224" = 4.25
  dimension "d225" = 4.25
  dimension "d226" = 20
  dimension "d227" = 20
  dimension "d234" = 2.93
  dimension "d235" = 4.25
  dimension "d236" = 20
  dimension "d237" = 2.93
  dimension "d238" = 4.25
  dimension "d239" = 20
  measures "d222" diameter of A0
  measures "d223" diameter of A1
  measures "d224" distance of A0.centre L0
  measures "d225" distance of A1.centre L0
  measures "d226" distance of A0.centre L1
  measures "d227" distance of A1.centre L2
  measures "d234" diameter of A2
  measures "d235" distance of A2.centre L6
  measures "d236" distance of A2.centre L7
  measures "d237" diameter of A3
  measures "d238" distance of A3.centre L8
  measures "d239" distance of A3.centre L9
extrude "Extrude8" cut sketch "Sketch6" against normal blind 103 contours A0 | A1 | A2 | A3 bodies 1
sketch "Sketch7" plane through (0, 0, 0) normal (-1, 0, 0) x (0, -1, 0)
  line L0 (-91.5, 15.5) -> (-91.5, 98)
  line L1 (-91.5, 98) -> (-8.5, 98)
  line L2 (-8.5, 98) -> (-8.5, 15.5)
  line L3 (-8.5, 15.5) -> (-91.5, 15.5)
  line L4 (-91.5, 7) -> (-8.5, 7)
  line L5 (-8.5, 7) -> (-8.5, 0)
  line L6 (-8.5, 0) -> (0, 0)
  line L7 (0, 0) -> (0, 113.5)
  line L8 (0, 113.5) -> (-8.5, 113.5)
  line L9 (-8.5, 113.5) -> (-8.5, 106.5)
  line L10 (-8.5, 106.5) -> (-91.5, 106.5)
  line L11 (-91.5, 106.5) -> (-91.5, 113.5)
  line L12 (-91.5, 113.5) -> (-100, 113.5)
  line L13 (-100, 113.5) -> (-100, 0)
  line L14 (-100, 0) -> (-91.5, 0)
  line L15 (-91.5, 0) -> (-91.5, 7)
  circle A0 centre (-76.5, 102.25) radius 1.465
  circle A1 centre (-23.5, 102.25) radius 1.465
  circle A2 centre (-76.5, 11.25) radius 1.465
  circle A3 centre (-23.5, 11.25) radius 1.465
  dimension "d248" = 2.93
  dimension "d249" = 4.25
  dimension "d250" = 23.5
  dimension "d251" = 2.93
  dimension "d252" = 4.25
  dimension "d253" = 23.5
  dimension "d254" = 2.93
  dimension "d255" = 4.25
  dimension "d256" = 23.5
  dimension "d257" = 2.93
  dimension "d258" = 4.25
  dimension "d259" = 23.5
  measures "d248" diameter of A0
  measures "d249" distance of L10 A0.centre
  measures "d250" distance of L13 A0.centre
  measures "d251" diameter of A1
  measures "d252" distance of L10 A1.centre
  measures "d253" distance of L7 A1.centre
  measures "d254" diameter of A2
  measures "d255" distance of L3 A2.centre
  measures "d256" distance of L13 A2.centre
  measures "d257" diameter of A3
  measures "d258" distance of L3 A3.centre
  measures "d259" distance of L7 A3.centre
extrude "Extrude9" cut sketch "Sketch7" against normal blind 100 contours A0 | A1 | A2 | A3 bodies 1
sketch "Sketch8" plane through (0, 0, 0) normal (0, 1, 0) x (1, 0, 0)
  circle A0 centre (23.5, -102.25) radius 1.465
  line L0 (91.5, -106.5) -> (8.5, -106.5)
  line L1 (0, 0) -> (0, -113.5)
  circle A1 centre (76.5, -102.25) radius 1.465
  line L2 (100, 0) -> (100, -113.5)
  circle A2 centre (23.5, -11.25) radius 1.465
  line L3 (91.5, -7) -> (8.5, -7)
  circle A3 centre (76.5, -11.25) radius 1.465
  dimension "d265" = 2.93
  dimension "d266" = 4.25
  dimension "d267" = 23.5
  dimension "d268" = 2.93
  dimension "d269" = 4.25
  dimension "d270" = 23.5
  dimension "d271" = 2.93
  dimension "d272" = 4.25
  dimension "d273" = 23.5
  dimension "d274" = 2.93
  dimension "d275" = 4.25
  dimension "d276" = 23.5
  measures "d265" diameter of A0
  measures "d266" distance of A0.centre L0
  measures "d267" distance of A0.centre L1
  measures "d268" diameter of A1
  measures "d269" distance of L0 A1.centre
  measures "d270" distance of A1.centre L2
  measures "d271" diameter of A2
  measures "d272" distance of A2.centre L3
  measures "d273" distance of L1 A2.centre
  measures "d274" diameter of A3
  measures "d275" distance of L3 A3.centre
  measures "d276" distance of L2 A3.centre
extrude "Extrude10" cut sketch "Sketch8" along normal blind 115 bodies 1
fillet "Fillet1" radius 1 20 edges at (95.75, 0, 113.5) (100, 4.25, 113.5) (100, 0, 56.75) (95.75, 8.5, 113.5) (91.5, 4.25, 113.5) (4.25, 8.5, 113.5) (8.5, 4.25, 113.5) (4.25, 0, 113.5) (0, 4.25, 113.5) (4.25, 91.5, 113.5) (0, 95.75, 113.5) (4.25, 100, 113.5) (8.5, 95.75, 113.5) (91.5, 95.75, 113.5) (95.75, 100, 113.5) (100, 95.75, 113.5) (95.75, 91.5, 113.5) (0, 0, 56.75) (100, 100, 56.75) (0, 100, 56.75) on bodies 1
fillet "Fillet2" radius 1 20 edges at (95.75, 91.5, 0) (91.5, 95.75, 0) (100, 95.25, 0) (99.7071, 99.7071, 0) (95.25, 100, 0) (4.25, 91.5, 0) (8.5, 95.75, 0) (0, 95.25, 0) (0.2929, 99.7071, 0) (4.75, 100, 0) (0, 4.75, 0) (0.2929, 0.2929, 0) (4.75, 0, 0) (4.25, 8.5, 0) (8.5, 4.25, 0) (95.75, 8.5, 0) (100, 4.75, 0) (99.7071, 0.2929, 0) (95.25, 0, 0) (91.5, 4.25, 0) on bodies 1

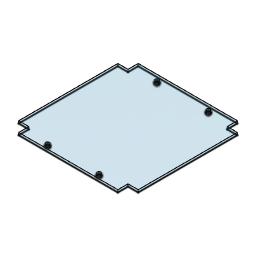
design "стенка"
Autodesk Fusion 360 part; units mm, degrees